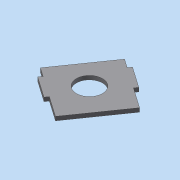
# Autodesk Inventor part: Part6
Saved by Autodesk Inventor 2016 SP1 (Build 200210100, 210)
## iProperties
Created: 2016-03-24
Part Number: Part6
Material: Generic
Document SubType Name: Modeling
Designer: Mohamed A.
Density: 1 g/cm^3
Appearance: Default
Author: Mohamed A.
Autodesk Inventor part; units mm, degrees
ref_plane "YZ Plane" through (0, 0, 0) normal (1, 0, 0) x (0, 1, 0)
ref_plane "XZ Plane" through (0, 0, 0) normal (0, 1, 0) x (-1, 0, 0)
ref_plane "XY Plane" through (0, 0, 0) normal (0, 0, 1) x (1, 0, 0)
sketch "Sketch1" plane through (0, 0, 0) normal (0, 0, 1) x (1, 0, 0)
  circle A0 centre (11.8, 0) radius 10.15 projected
  line L0 (0.848, -26.1294) -> (7.0019, -30.4166) projected
  line L1 (7.0019, -30.4166) -> (8.7168, -27.9551) projected
  line L2 (-11.9996, -17.1789) -> (-6.1263, -21.2706) projected
  line L3 (-6.1263, -21.2706) -> (-4.4115, -18.8091) projected
  line L4 (-4.4115, -18.8091) -> (-2.1551, -20.381) projected
  line L5 (-2.1551, -20.381) -> (-1.0118, -18.74) projected
  line L6 (-1.0118, -18.74) -> (-1.9554, -18.0826) projected
  line L7 (-1.9554, -18.0826) -> (-0.5835, -16.1134) projected
  line L8 (-0.5835, -16.1134) -> (0.3601, -16.7708) projected
  line L9 (0.3601, -16.7708) -> (0.7031, -16.2785) projected
  line L10 (0.7031, -16.2785) -> (3.1646, -17.9933) projected
  line L11 (3.1646, -17.9933) -> (2.8216, -18.4856) projected
  line L12 (2.8216, -18.4856) -> (3.7652, -19.143) projected
  line L13 (3.7652, -19.143) -> (2.3933, -21.1123) projected
  line L14 (2.3933, -21.1123) -> (1.4497, -20.4549) projected
  line L15 (1.4497, -20.4549) -> (0.3065, -22.0959) projected
  line L16 (0.3065, -22.0959) -> (2.5629, -23.6679) projected
  line L17 (2.5629, -23.6679) -> (0.848, -26.1294) projected
  line L18 (8.7168, -27.9551) -> (18.3578, -34.6717) projected
  line L19 (18.3578, -34.6717) -> (46.5961, 5.8617) projected
  line L20 (46.5961, 5.8617) -> (36.9551, 12.5783) projected
  line L21 (36.9551, 12.5783) -> (38.67, 15.0399) projected
  line L22 (38.67, 15.0399) -> (32.5161, 19.3271) projected
  line L23 (32.5161, 19.3271) -> (30.8012, 16.8655) projected
  line L24 (30.8012, 16.8655) -> (28.5448, 18.4375) projected
  line L25 (28.5448, 18.4375) -> (27.4015, 16.7965) projected
  line L26 (27.4015, 16.7965) -> (28.3451, 16.1391) projected
  line L27 (28.3451, 16.1391) -> (26.9732, 14.1699) projected
  line L28 (26.9732, 14.1699) -> (26.0296, 14.8272) projected
  line L29 (26.0296, 14.8272) -> (25.6867, 14.3349) projected
  line L30 (25.6867, 14.3349) -> (23.2251, 16.0498) projected
  line L31 (23.2251, 16.0498) -> (23.5681, 16.5421) projected
  line L32 (23.5681, 16.5421) -> (22.6245, 17.1995) projected
  line L33 (22.6245, 17.1995) -> (23.9964, 19.1687) projected
  line L34 (23.9964, 19.1687) -> (24.94, 18.5114) projected
  line L35 (24.94, 18.5114) -> (26.0833, 20.1524) projected
  line L36 (26.0833, 20.1524) -> (23.8268, 21.7244) projected
  line L37 (23.8268, 21.7244) -> (25.5417, 24.1859) projected
  line L38 (25.5417, 24.1859) -> (19.6685, 28.2776) projected
  line L39 (19.6685, 28.2776) -> (17.9536, 25.8161) projected
  line L40 (17.9536, 25.8161) -> (8.0319, 32.7281) projected
  line L41 (8.0319, 32.7281) -> (-20.2064, -7.8053) projected
  line L42 (-20.2064, -7.8053) -> (-10.2847, -14.7174) projected
  line L43 (-10.2847, -14.7174) -> (-11.9996, -17.1789) projected
  point P0 (0, 0)
extrude "Extrusion1" add sketch "Sketch1" along normal blind 3
body "Solid1"
